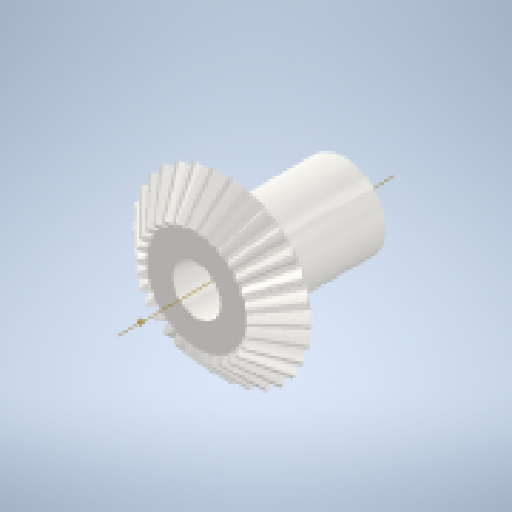
# Autodesk Inventor part: Bevel Gear2
Saved by Autodesk Inventor 2023 (Build 270158000, 158)
## iProperties
Created: 2023-02-13
Part Number: Bevel Gear2
Material: Steel, Mild
Document SubType Name: Modeling
Designer: deepa
Categories: <?xml version="1.0" encoding="UTF-16"?> <MemberInstance><Categories><FamilyTemplate><FamilyTemplateParameter ValueType="xs:double" Id="1" ObjectReferenceKey="da_z" ObjectType="kUserParameterObject"/><FamilyTemplateParameter ValueType="xs:double" Id="2" ObjectReferenceKey="da_b" ObjectType="kUserParameterObject"/><FamilyTemplateParameter ValueType="xs:double" Id="3" ObjectReferenceKey="da_beta" ObjectType="kUserParameterObject"/><FamilyTemplateParameter ValueType="xs:double" Id="4" ObjectReferenceKey="da_dae" ObjectType="kUserParameterObject"/><FamilyTemplateParameter ValueType="xs:double" Id="5" ObjectReferenceKey="da_ve" ObjectType="kUserParameterObject"/><FamilyTemplateParameter ValueType="xs:double" Id="6" ObjectReferenceKey="da_omega" ObjectType="kUserParameterObject"/><FamilyTemplateParameter ValueType="xs:string" Id="7" ObjectReferenceKey="EAIAABAAAAAAHwAAAAAAAIAAAAAAAAAA" ObjectType="83914240" SubObjectId="SurfaceGeometry"/></FamilyTemplate><ParamToTemplateMap><ParamToTemplate CategoryParameter="//CategoryParameter[@InternalName='046C89C9-8512-4d59-83FE-43B91F4F132A']" TemplateParameter="1"/><ParamToTemplate CategoryParameter="//CategoryParameter[@InternalName='2552DF32-E462-4b46-AEBF-C6C7768E72AC']" TemplateParameter="2"/><ParamToTemplate CategoryParameter="//CategoryParameter[@InternalName='C9EE641D-15FC-4fae-A226-E94C4372FDD7']" TemplateParameter="3"/><ParamToTemplate><ParamToTemplate CategoryParameter="//CategoryParameter[@InternalName='00B6519A-459B-49c7-AD84-2E56D39A5744']" ConstantValue="-0.000000"/></ParamToTemplate><ParamToTemplate><ParamToTemplate CategoryParameter="//CategoryParameter[@InternalName='04B31F0E-C7A6-4894-AA32-9629BEFACF47']" ConstantValue="1.000000"/></ParamToTemplate><ParamToTemplate><ParamToTemplate CategoryParameter="//CategoryParameter[@InternalName='43CBEC2E-7847-49e7-A936-2F7889FCB2D9']" ConstantValue="0.200000"/></ParamToTemplate><ParamToTemplate><ParamToTemplate CategoryParameter="//CategoryParameter[@InternalName='B1EFC894-105D-4ebd-86BF-FA20ED196853']" ConstantValue="0.300000"/></ParamToTemplate><ParamToTemplate><ParamToTemplate CategoryParameter="//CategoryParameter[@InternalName='51175063-3D10-4879-93E8-6246FE8B403D']" ConstantValue="2060000000.000000"/></ParamToTemplate><ParamToTemplate><ParamToTemplate CategoryParameter="//CategoryParameter[@InternalName='A3A52E27-4454-46a9-B0BD-C932399B70AF']" ConstantValue="0.300000"/></ParamToTemplate><ParamToTemplate CategoryParameter="//CategoryParameter[@InternalName='2A200944-5A8C-41ca-B96E-8520D2E510F1']" TemplateParameter="4"/><ParamToTemplate><ParamToTemplate CategoryParameter="//CategoryParameter[@InternalName='1A637F62-92C8-44bc-B81F-10802510B579']" ConstantValue="2.935076"/></ParamToTemplate><ParamToTemplate CategoryParameter="//CategoryParameter[@InternalName='B52DD4BE-6863-48fb-BF58-89EF6F9EC65C']" TemplateParameter="5"/><ParamToTemplate><ParamToTemplate CategoryParameter="//CategoryParameter[@InternalName='3956BFF2-84D2-457d-93C2-9B0613DEBA67']" ConstantValue="1.335406"/></ParamToTemplate><ParamToTemplate CategoryParameter="//CategoryParameter[@InternalName='739CFA02-461B-4bf8-8049-181FCAD8B28F']" TemplateParameter="6"/><ParamToTemplate><ParamToTemplate CategoryParameter="//CategoryParameter[@InternalName='A27E999F-E2CE-4481-8A2A-EBF499C4C3C5']" ConstantValue="-0.000000"/></ParamToTemplate><ParamToTemplate><ParamToTemplate CategoryParameter="//CategoryParameter[@InternalName='9E1B4470-B2D3-4ff1-B813-535BB4CDF51A']" ConstantValue="3520000.000000"/></ParamToTemplate><ParamToTemplate><ParamToTemplate CategoryParameter="//CategoryParameter[@InternalName='F8452263-BFF6-458c-9FB1-07C4B99E95CD']" ConstantValue="11400000.000000"/></ParamToTemplate><ParamToTemplate><ParamToTemplate CategoryParameter="//CategoryParameter[@InternalName='3E3BB259-FD49-497f-8171-6EBC954A3479']" ConstantValue="2.000000"/></ParamToTemplate><ParamToTemplate CategoryParameter="//CategoryParameter[@InternalName='27C3BAF2-7550-4e4b-AE2C-0DB134B7D9B7']" TemplateParameter="7"/></ParamToTemplateMap><Category DisplayName="Gear" InternalName="DC85795E-93AB-48d5-8EEE-5A27447B64BD" Mnemonic="Gear"><CategoryParameter DisplayName="z" InternalName="046C89C9-8512-4d59-83FE-43B91F4F132A" Mnemonic="z"/><CategoryParameter DisplayName="b" InternalName="2552DF32-E462-4b46-AEBF-C6C7768E72AC" Mnemonic="b"/><CategoryParameter DisplayName="||b|" InternalName="C9EE641D-15FC-4fae-A226-E94C4372FDD7" Mnemonic="beta"/><CategoryParameter DisplayName="x" InternalName="00B6519A-459B-49c7-AD84-2E56D39A5744" Mnemonic="x"/><CategoryParameter DisplayName="a*" InternalName="04B31F0E-C7A6-4894-AA32-9629BEFACF47" Mnemonic="a"/><CategoryParameter DisplayName="c*" InternalName="43CBEC2E-7847-49e7-A936-2F7889FCB2D9" Mnemonic="c"/><CategoryParameter DisplayName="r|.f|*" InternalName="B1EFC894-105D-4ebd-86BF-FA20ED196853" Mnemonic="rf"/><CategoryParameter DisplayName="E" InternalName="51175063-3D10-4879-93E8-6246FE8B403D" Mnemonic="E"/><CategoryParameter DisplayName="||m|" InternalName="A3A52E27-4454-46a9-B0BD-C932399B70AF" Mnemonic="mi"/><Category DisplayName="BevelGear" InternalName="0C98F69A-0C2B-4791-B2FE-7691BB227E77" Mnemonic="BevelGear"><CategoryParameter DisplayName="d|.ae|" InternalName="2A200944-5A8C-41ca-B96E-8520D2E510F1" Mnemonic="dae"/><CategoryParameter DisplayName="d|.ai|" InternalName="1A637F62-92C8-44bc-B81F-10802510B579" Mnemonic="dai"/><CategoryParameter DisplayName="A|.e|" InternalName="B52DD4BE-6863-48fb-BF58-89EF6F9EC65C" Mnemonic="ve"/><CategoryParameter DisplayName="A|.i|" InternalName="3956BFF2-84D2-457d-93C2-9B0613DEBA67" Mnemonic="vi"/><CategoryParameter DisplayName="||S|" InternalName="739CFA02-461B-4bf8-8049-181FCAD8B28F" Mnemonic="omega"/><CategoryParameter DisplayName="x|.t|" InternalName="A27E999F-E2CE-4481-8A2A-EBF499C4C3C5" Mnemonic="xt"/><CategoryParameter DisplayName="||s||.Flim|" InternalName="9E1B4470-B2D3-4ff1-B813-535BB4CDF51A" Mnemonic="sFlim"/><CategoryParameter DisplayName="||s||.Hlim|" InternalName="F8452263-BFF6-458c-9FB1-07C4B99E95CD" Mnemonic="sHlim"/><CategoryParameter DisplayName="type" InternalName="3E3BB259-FD49-497f-8171-6EBC954A3479" Mnemonic="type"/><CategoryParameter DisplayName="PitchDiameter" InternalName="27C3BAF2-7550-4e4b-AE2C-0DB134B7D9B7" Mnemonic="IDS_PITCHDIAM"/></Category></Category></Categories></MemberInstance>
Mass: 60.9118 g
Surface Area: 34.3074 cm^2
Volume: 7.7496 cm^3
Density: 7.86 g/cm^3
Appearance: Steel
CustomPartVersion: 1
Author: deepa
Autodesk Inventor part; units mm, degrees
ref_plane "Mesh Plane2" through (0, 0, 0) normal (0.9945219, 0.1045285, 0) x (0, 0, 1)
sketch "Teeth Body Sketch" plane through (0, 0, 0) normal (1, 0, 0) x (0, 1, 0)
  line L0 (0, 0) -> (21.227208, -23.772792) construction
  line L1 (21.227208, -23.772792) -> (23.56066, -21.43934)
  line L2 (23.56066, -21.43934) -> (0, 0) construction
  line L3 (22.5, -22.5) -> (0, 0) construction
  line L4 (13.221926, -14.807511) -> (14.675379, -13.354058)
  line L5 (21.227208, -23.772792) -> (13.221926, -14.807511)
  line L6 (23.56066, -21.43934) -> (14.675379, -13.354058)
  line L7 (0, -39.386751) -> (0, 6.564458)
  line L8 (0, -22.5) -> (23.56066, -22.5) construction
  dimension "d0" = 45
  dimension "d1" = 42.45442
  dimension "d2" = 47.12132
  dimension "d3" = 12
  dimension "d4" = 21.43934
  constraints: 16 end point, 4 point on line, 3 perpendicular, 2 collinear, 1 horizontal alignment, 1 vertical alignment
  measures "d0" diameter of L3.start L7
  measures "d1" diameter of L0.end L7
  measures "d2" diameter of L1.end L7
  measures "d3" distance between parallel lines of L1 L4
  measures "d4" vertical distance of L1.end L0.start
revolve "Teeth Body" add sketch "Teeth Body Sketch" angle 360 about axis through (0, 0, 0) along (0, 0, 1)
ref_plane "Tooth Plane" through (0, 22.5, -22.5) normal (0, -0.7071068, 0.7071068) x (1, 0, 0)
sketch "Start Sketch" plane through (0, 22.5, -22.5) normal (0, -0.7071068, 0.7071068) x (1, 0, 0)
  line L0 (0, -23.505131) -> (0, 10.644758)
  arc A0 (-0.554831, -2.196) -> (-2.53053, 2.396553) centre (-11.758562, -4.294557) ccw
  arc A1 (2.53053, 2.396553) -> (0.554831, -2.196) centre (11.758562, -4.294557) ccw
  line L1 (-0.554831, -2.196) -> (0.554831, -2.196)
  arc A2 (2.53053, 2.396553) -> (-2.53053, 2.396553) centre (0, -31.819805) ccw
  dimension "d7" = 11.39858
  dimension "d8" = 11.75856
  dimension "d9" = 27.52525
  dimension "d57" = 34.30981
  dimension "d58" = 29.62381
  constraints: 6 point on circle, 3 centre point, 3 symmetric about line, 2 end point, 1 coincident, 1 perpendicular, 1 other
  measures "d7" radius of A0
  measures "d8" horizontal distance of point (0, -31.82) A0.centre
  measures "d9" vertical distance of point (0, -31.82) A0.centre
  measures "d57" radius of A2
  measures "d58" distance from line of A2.centre L1
sketch "End Sketch" plane through (0, 13.898046, -13.898046) normal (0, -0.7071068, 0.7071068) x (1, 0, 0)
  line L0 (0, -15.35404) -> (0, 6.953444)
  arc A0 (-0.342714, -1.356449) -> (-1.563085, 1.480329) centre (-7.263157, -2.652709) ccw
  arc A1 (1.563085, 1.480329) -> (0.342714, -1.356449) centre (7.263157, -2.652709) ccw
  line L1 (-0.342714, -1.356449) -> (0.342714, -1.356449)
  arc A2 (1.563085, 1.480329) -> (-1.563085, 1.480329) centre (0, -19.654805) ccw
  dimension "d12" = 7.0408
  dimension "d15" = 7.26316
  dimension "d16" = 17.0021
  dimension "d59" = 21.19286
  dimension "d60" = 18.29836
  constraints: 6 point on circle, 3 centre point, 3 symmetric about line, 2 end point, 1 coincident, 1 other
  measures "d12" radius of A0
  measures "d15" horizontal distance of A0.centre point (0, -19.655)
  measures "d16" vertical distance of A0.centre point (0, -19.655)
  measures "d59" radius of A2
  measures "d60" distance from line of A2.centre L1
loft "Loft" cut profiles "Start Sketch", "End Sketch"
pattern_circular "Circular Pattern" count 30 over 360 about axis through (0, 0, 0) along (0, 0, 1) of "Loft"
ref_plane "End Plane" through (0, 13.898046, -13.898046) normal (0, -0.7071068, 0.7071068) x (1, 0, 0)
sketch3d "3D Sketch Right"
ref_plane "End Plane Right" through (-3.337554, 13.491346, -13.898046) normal (0.1698085, -0.6864146, 0.7071068) x (0.9707369, 0.2401456, 0)
sketch "End Sketch Right" plane through (-3.337554, 13.491346, -13.898046) normal (0.1698085, -0.6864146, 0.7071068) x (0.9707369, 0.2401456, 0)
  arc A0 (-0.342714, -1.356449) -> (-1.563085, 1.480329) centre (-7.263157, -2.652709) ccw
  line L0 (0, -27.380033) -> (0, 11.491883)
  arc A1 (1.563085, 1.480329) -> (0.342714, -1.356449) centre (7.263157, -2.652709) ccw
  line L1 (-0.342714, -1.356449) -> (0.342714, -1.356449)
  arc A2 (1.563085, 1.480329) -> (-1.563085, 1.480329) centre (0, -19.654805) ccw
  dimension "d70" = 7.26316
  dimension "d71" = 17.0021
  dimension "d72" = 7.0408
  dimension "d73" = 18.29836
  dimension "d74" = 21.19286
  constraints: 6 point on circle, 3 centre point, 3 symmetric about line, 2 end point, 1 coincident, 1 perpendicular, 1 other
  measures "d70" horizontal distance of A2.centre A0.centre
  measures "d71" vertical distance of point (0, -19.655) A0.centre
  measures "d72" radius of A0
  measures "d73" distance from line of point (0, -19.655) L1
  measures "d74" radius of A2
feature "Loft Right" [suppressed]
pattern_circular "Circular Pattern Right" [suppressed]
sketch3d "3D Sketch Left"
ref_plane "End Plane Left" through (3.34776, 13.491346, -13.902013) normal (-0.1702885, -0.6862561, 0.7071452) x (0.9705655, -0.2408374, 0)
sketch "End Sketch Left" plane through (3.34776, 13.491346, -13.902013) normal (-0.1702885, -0.6862561, 0.7071452) x (0.9705655, -0.2408374, 0)
  line L0 (0, -31.789523) -> (0, 14.7668)
  arc A0 (-0.342714, -1.35538) -> (-1.563085, 1.481398) centre (-7.263157, -2.651639) ccw
  arc A1 (1.563085, 1.481398) -> (0.342714, -1.35538) centre (7.263157, -2.651639) ccw
  line L1 (-0.342714, -1.35538) -> (0.342714, -1.35538)
  ellipse E0 centre (0, -9.442232) end of major axis (14.675379, -9.442232) minor radius 10.377624
  arc A2 (1.563085, 1.481398) -> (-1.563085, 1.481398) centre (0, -19.653736) ccw
  dimension "d56" = 10.37762
  dimension "d30" = 7.0408
  dimension "d31" = 7.26316
  dimension "d32" = 17.0021
  dimension "d61" = 21.19286
  dimension "d62" = 18.29836
  constraints: 6 point on circle, 3 centre point, 3 symmetric about line, 2 end point, 1 coincident, 2 other
  measures "d30" radius of A0
  measures "d31" horizontal distance of point (0, -19.654) A0.centre
  measures "d32" vertical distance of A0.centre point (0, -19.654)
  measures "d61" radius of A2
  measures "d62" distance from line of point (0, -19.654) L1
feature "Loft Left" [suppressed]
pattern_circular "Circular Pattern Left" [suppressed]
sketch "Body Sketch" plane through (0, 0, 0) normal (1, 0, 0) x (0, 1, 0)
  line L0 (0, -35.037536) -> (0, -19.530831)
  line L1 (21.227208, -23.772792) -> (13.221926, -14.807511)
  line L2 (13.221926, -14.807511) -> (0, -14.807511)
  line L3 (21.227208, -23.772792) -> (0, -23.772792)
  constraints: 4 end point, 2 perpendicular, 2 point on line
sketch "Body Sketch outline for Fix Body" plane through (0, 0, 0) normal (1, 0, 0) x (0, 1, 0)
  line L0 (0, -23.772792) -> (21.227208, -23.772792)
  line L1 (0, -14.807511) -> (0, -23.772792)
  line L2 (13.221926, -14.807511) -> (0, -14.807511)
  line L3 (21.227208, -23.772792) -> (13.221926, -14.807511)
revolve "Fix Body" add sketch "Body Sketch outline for Fix Body" angle 360 about axis through (0, 0, 0) along (0, 0, 1)
sketch "Sketch6" plane through (0, 0, 0) normal (1, 0, 0) x (0, 1, 0)
  line L0 (22.5, -22.5) -> (0, 0)
  line L1 (0, -37.799919) -> (0, 6.299986)
surface revolve "Pitch Diameter" sketch "Sketch6" angle 360 about axis through (0, 0, 0) along (0, 0, 1) shown no curves L0
sketch "Sketch8" plane through (0, 0, -23.772792) normal (0, 0, -1) x (-1, 0, 0)
  circle A0 centre (0, 0) radius 11
  dimension "d94" = 22
  constraints: 1 centre point, 1 coincident
  measures "d94" diameter of A0
extrude "Extrusion1" add sketch "Sketch8" along normal blind 18
sketch "Sketch9" plane through (0, 0, -41.772792) normal (0, 0, -1) x (-1, 0, 0)
  circle A0 centre (0, 0) radius 6.35
  dimension "d97" = 12.7
  constraints: 1 centre point, 1 coincident
  measures "d97" diameter of A0
extrude "Extrusion2" cut sketch "Sketch9" against normal blind 40
ref_plane "Work Plane6" through (0, 0, 0) normal (0.1045285, 0.9945219, 0) x (0.9945219, -0.1045285, 0)
sketch "Sketch10" plane through (0, 0, 0) normal (0.1045285, 0.9945219, 0) x (0.9945219, -0.1045285, 0)
  circle A0 centre (0, 33.772792) radius 3.25
  line L0 (11, 41.772792) -> (-11, 41.772792)
  point P0 (0, 0)
  dimension "d100" = 6.5
  dimension "d101" = 8
  constraints: 1 centre point
  measures "d100" diameter of A0
  measures "d101" distance from line of A0.centre L0
extrude "Extrusion3" cut sketch "Sketch10" against normal blind 11
sketch "Sketch11" plane through (0, 0, -23.772792) normal (0, 0, -1) x (-1, 0, 0)
  point P0 (0, 0)
equation "\"d0\" = da_de"
equation "\"d1\" = da_dfe"
equation "\"d2\" = da_dae"
equation "\"d3\" = da_b"
equation "\"d4\" = da_ve"
equation "\"d7\" = fd_rr"
equation "\"d8\" = fd_x"
equation "\"d9\" = fd_y"
equation "\"d57\" = 0.5 * fd_dva + 0.3 * da_he"
equation "\"d58\" = 0.5 * fd_dva - 1.12 * da_he"
equation "\"da_teethtype\" = 0"
equation "\"da_b\" = 12"
equation "\"da_de\" = 45"
equation "\"da_dae\" = 47.12132"
equation "\"da_dfe\" = 42.45442"
equation "\"da_le\" = 31.81981"
equation "\"da_omega\" = 90deg"
equation "\"da_beta\" = 0"
equation "\"da_delta\" = 45deg"
equation "\"da_alpha\" = 20deg"
equation "\"da_he\" = 3.3"
equation "\"da_ve\" = 21.43934"
equation "\"da_zv\" = 42.426407"
equation "\"fd_loft\" = da_b + 0.05 * da_he"
equation "\"fd_x\" = fd_x1 + fd_x2"
equation "\"fd_y\" = fd_y1 - fd_y2"
equation "\"fd_dd\" = fd_dva - 0.8 * da_he"
equation "\"da_dvw\" = 63.63961"
equation "\"d11\" = fd_loft"
equation "\"da_dm\" = 36.51472"
equation "\"da_x\" = 0"
equation "\"da_m\" = 1.5"
equation "\"d50\" = da_omega"
equation "\"fd_rr\" = 11.398576"
equation "\"fd_dva\" = 66.63961"
equation "\"fd_x1\" = 1.190909"
equation "\"fd_x2\" = 10.567653"
equation "\"fd_y1\" = 31.797511"
equation "\"fd_y2\" = 4.272263"
body "Solid1"
body "Srf1"
